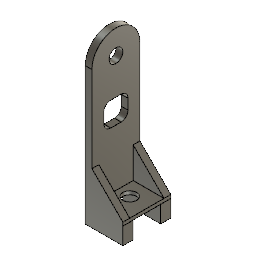
final_gear_mount v11 (Autodesk Fusion 360 design; units mm, degrees)
Autodesk Fusion 360 part; units mm, degrees
note: some values were not read from the file. Set by a fixed rule: which sketch regions a step uses.
sketch "Sketch1" plane through (0, 0, 0) normal (0, 0, 1) x (1, 0, 0)
  line L0 (0, 0) -> (11, 0)
  line L1 (11, 0) -> (11, 5)
  line L2 (11, 5) -> (0, 5)
  line L3 (0, 5) -> (0, 0)
  line L4 (1, 5) -> (10, 5)
  line L5 (10, 5) -> (10, 1)
  line L6 (10, 1) -> (1, 1)
  line L7 (1, 1) -> (1, 5)
  dimension "d1" = 1
  dimension "d2" = 1
  dimension "d3" = 1
  dimension "d4" = 9
  dimension "d5" = 4
  constraint horizontal L0
  constraint vertical L1
  constraint horizontal L2
  constraint vertical L3
  constraint coincident L0.start L3.end
  constraint horizontal L4
  constraint vertical L5
  constraint horizontal L6
  constraint vertical L7
  constraint coincident L2 L4.start
  measures "d1" distance of L3 L7
  measures "d2" distance of L1 L5
  measures "d3" distance of L0 L6
  measures "d4" distance of L5 L7
  measures "d5" distance of L2 L6
extrude "Extrude1" add sketch "Sketch1" along normal blind 95.39 contours L0 L1 L2 L3 L5 L6 L7
sketch "Sketch2" plane through (0, 1, 0) normal (0, 1, 0) x (-1, 0, 0)
  line L0 (-10, 0) -> (-1, 0)
  line L1 (-1, 0) -> (-1, 95.39)
  line L2 (-1, 95.39) -> (-10, 95.39)
  line L3 (-10, 95.39) -> (-10, 0)
  line L4 (0, 0) -> (-11, 0)
  line L5 (-11, 0) -> (-11, 1)
  line L6 (-11, 1) -> (0, 1)
  line L7 (0, 1) -> (0, 0)
  dimension "d8" = 1
  constraint horizontal L4
  constraint vertical L5
  constraint horizontal L6
  constraint vertical L7
  constraint coincident L4.start L7.end
  measures "d8" distance of L4 L6
extrude "Extrude2" add sketch "Sketch2" along normal blind 6 from surface at 4 contours L0 L1 L3 L4 L6 | L3 L4 L5 L6 | L1 L4 L6 L7
extrude "Extrude3" add 1 faces at (7, 5, 0.6667) along direction (0, -1, 0) up to surface (4 mm away)
sketch "Sketch3" plane through (0, 0, 1) normal (0, 0, 1) x (-1, 0, 0)
  line L0 (-10, -5) -> (-11, -5)
  line L1 (-11, -5) -> (-11, -11)
  line L2 (-11, -11) -> (0, -11)
  line L3 (0, -11) -> (0, -5)
  line L4 (0, -5) -> (-1, -5)
  line L5 (-1, -5) -> (-1, -1)
  line L6 (-1, -1) -> (-10, -1)
  line L7 (-10, -1) -> (-10, -5)
  line L8 (0, -7.5) -> (-11, -7.5)
  circle A0 centre (-5.5, -7.5) radius 2
  circle A1 centre (-5.5, -7.5) radius 3.5
  line L9 (0, -7.5) -> (-11, -7.5)
  line L10 (-11, -7.5) -> (-11, -14)
  line L11 (-11, -14) -> (0, -14)
  line L12 (0, -14) -> (0, -7.5)
  line L13 (-5.5, -7.5) -> (-5.5, -11)
  line L14 (-5.5, -11) -> (-5.5, -14)
  point P0 (-2, -7.5)
  dimension "d14" = 4
  dimension "d15" = 7
  dimension "d17" = 3
  dimension "d32" = 6.5
  constraint coincident L3 L8.start
  constraint coincident L1 L8.end
  constraint perpendicular L1 L8
  constraint midpoint L8 A0.centre
  constraint concentric A0 A1
  constraint coincident L8 P0
  constraint coincident A1 P0
  constraint horizontal L9
  constraint vertical L10
  constraint horizontal L11
  constraint vertical L12
  constraint coincident A0.centre A1.centre
  constraint coincident A1 L13.end
  constraint perpendicular L2 L13
  constraint midpoint L11 L14.end
  constraint perpendicular L11 L14
  measures "d14" diameter of A0
  measures "d15" diameter of A1
  measures "d17" distance of L13.end L14.end
  measures "d32" distance of L6 L9
extrude "Extrude4" add sketch "Sketch3" against normal up to surface (1 mm away) contours L1 L2 L8 A1 L9 L10 | L2 L10 L11 L14 | L2 L3 L8 A1 L9 L12 | L2 L11 L12 L14
extrude "Extrude5" cut sketch "Sketch3" against normal blind 5 contours L8 A0 L9 | L8 A0 L9 L13 | L8 A0 L9 L13
sketch "Sketch4" plane through (0, 0, 0) normal (-1, 0, 0) x (0, -1, 0)
  line L0 (-14, 0) -> (0, 0)
  line L1 (0, 0) -> (0, 95.39)
  line L2 (0, 95.39) -> (-5, 95.39)
  line L3 (-5, 95.39) -> (-5, 1)
  line L4 (-5, 1) -> (-14, 1)
  line L5 (-14, 1) -> (-14, 0)
  line L6 (-14, 1) -> (-5, 10)
  line L7 (-14, 1) -> (-7.5, 1)
  dimension "d22" = 45
  constraint coincident L4.end L5.start
  constraint coincident L3 L6.end
  measures "d22" angle of L6 L7
extrude "Extrude6" add sketch "Sketch4" against normal up to surface (1 mm away) contours L3 L4 L6 L7
ref_plane "WorkPlane1" through (5.5, 0, 0) normal (1, 0, 0) x (0, 1, 0)
mirror "Mirror1" about plane through (5.5, 0, 0) normal (1, 0, 0) of "Extrude6"
sketch "Sketch5" plane through (0, 0, 0) normal (0, 0, -1) x (1, 0, 0)
  circle A0 centre (5.5, -7.5) radius 2
  line L0 (11, -14) -> (11, 0)
  line L1 (11, 0) -> (0, 0)
  line L2 (0, 0) -> (0, -14)
  line L3 (0, -14) -> (11, -14)
  line L4 (0, 0) -> (11, 0)
  line L5 (11, 0) -> (11, -3)
  line L6 (11, -3) -> (0, -3)
  line L7 (0, -3) -> (0, 0)
  line L8 (0, -14) -> (11, -14)
  line L9 (11, -14) -> (11, -11)
  line L10 (11, -11) -> (0, -11)
  line L11 (0, -11) -> (0, -14)
  dimension "d28" = 3
  dimension "d29" = 3
  constraint horizontal L4
  constraint vertical L5
  constraint horizontal L6
  constraint vertical L7
  constraint coincident L0 L5.end
  constraint coincident L1.end L2.start
  constraint horizontal L8
  constraint vertical L9
  constraint horizontal L10
  constraint vertical L11
  constraint coincident L0 L9.end
  constraint coincident L2.end L3.start
  measures "d28" distance of L2.end L10.end
  measures "d29" distance of L4 L6
extrude "Extrude7" add sketch "Sketch5" along normal blind 5 contours L0 L2 L3 L8 L9 L10 L11 | L0 L1 L2 L4 L5 L6 L7
sketch "Sketch6" plane through (11, 0, 0) normal (1, 0, 0) x (0, 1, 0)
  line L0 (0, 0) -> (3, 0)
  line L1 (3, 0) -> (11, 0)
  line L2 (11, 0) -> (14, 0)
  line L3 (14, 0) -> (14, 1)
  line L4 (14, 1) -> (5, 10)
  line L5 (5, 10) -> (5, 95.39)
  line L6 (5, 95.39) -> (0, 95.39)
  line L7 (0, 95.39) -> (0, 0)
  line L8 (14, 1) -> (-30, 1)
  line L9 (-30, 1) -> (-30, 130)
  line L10 (-30, 130) -> (14, 130)
  line L11 (14, 130) -> (14, 1)
  constraint horizontal L8
  constraint vertical L9
  constraint horizontal L10
  constraint vertical L11
  constraint coincident L3.end L4.start
extrude "Extrude8" cut sketch "Sketch6" against normal blind 100 contours L4 L5 L6 L7 L8
sketch "Sketch7" plane through (0, 0, 1) normal (0, 0, 1) x (-1, 0, 0)
  line L0 (-11, -14) -> (0, -14)
  line L1 (0, -14) -> (0, 0)
  line L2 (0, 0) -> (-11, 0)
  line L3 (-11, 0) -> (-11, -14)
  circle A0 centre (-5.5, -7.5) radius 2
  line L4 (0, -14) -> (-2, -14)
  line L5 (-2, -14) -> (-2, 0)
  line L6 (-2, 0) -> (0, 0)
  line L7 (0, 0) -> (0, -14)
  point P0 (0, -11)
  dimension "d35" = 2
  constraint horizontal L4
  constraint vertical L5
  constraint horizontal L6
  constraint vertical L7
  constraint coincident L2 L5.end
  constraint coincident L0.end L1.start
  measures "d35" distance of L5 P0
extrude "Extrude9" add sketch "Sketch7" along normal blind 41 contours L0 L1 L2 L4 L5 L6 L7
sketch "Sketch8" plane through (0, 0, 0) normal (-1, 0, 0) x (0, -1, 0)
  line L0 (-14, 42) -> (-14, -5)
  line L1 (-14, -5) -> (-11, -5)
  line L2 (-11, -5) -> (-11, 0)
  line L3 (-11, 0) -> (-3, 0)
  line L4 (-3, 0) -> (-3, -5)
  line L5 (-3, -5) -> (0, -5)
  line L6 (0, -5) -> (0, 42)
  line L7 (0, 42) -> (-14, 42)
  line L8 (-7, 42) -> (-7, 26)
  circle A0 centre (-7, 35) radius 7
  circle A1 centre (-7, 35) radius 2
  dimension "d38" = 4
  constraint midpoint L7 L8.start
  constraint perpendicular L7 L8
  constraint coincident L8 A0.centre
  constraint coincident L8.start A0
  constraint tangent L6 A0
  constraint concentric A0 A1
  measures "d38" diameter of A1
extrude "Extrude10" cut sketch "Sketch8" against normal blind 10 contours L0 L7 A0 | L6 L7 A0 | L8 A1 | L8 A1
sketch "Sketch9" plane through (2, 0, 0) normal (1, 0, 0) x (0, 1, 0)
  arc A0 (14, 35) -> (0, 35) centre (7, 35) ccw
  line L0 (0, 35) -> (0, 1)
  line L1 (0, 1) -> (14, 1)
  line L2 (14, 1) -> (14, 35)
  circle A1 centre (7, 35) radius 2
  line L3 (4.5, 18.5) -> (9.5, 18.5)
  line L4 (9.5, 18.5) -> (9.5, 22.5)
  line L5 (9.5, 22.5) -> (4.5, 22.5)
  line L6 (4.5, 22.5) -> (4.5, 18.5)
  line L7 (7, 22.5) -> (7, 35)
  dimension "d41" = 5
  dimension "d42" = 4
  dimension "d43" = 90
  dimension "d44" = 12.5
  constraint horizontal L3
  constraint vertical L4
  constraint horizontal L5
  constraint vertical L6
  constraint midpoint L5 L7.start
  constraint coincident A0.centre A1.centre
  measures "d41" distance of L3.start L3.end
  measures "d42" distance of L3.end L4.end
  measures "d43" angle of L5 L7
  measures "d44" distance of L7.start A0.centre
extrude "Extrude11" cut sketch "Sketch9" against normal blind 10 contours L3 L4 L5 L6
extrude "Extrude12" cut 1 faces at (1.3333, 7.8333, 22.5) along direction (0, 0, 1) blind 1
sketch "Sketch10" plane through (0, 0, 0) normal (-1, 0, 0) x (0, -1, 0)
  line L0 (-4.5, 23.5) -> (-4.5, 18.5)
  line L1 (-4.5, 18.5) -> (-9.5, 18.5)
  line L2 (-9.5, 18.5) -> (-9.5, 23.5)
  line L3 (-9.5, 23.5) -> (-4.5, 23.5)
  circle A0 centre (-7, 35) radius 2
  arc A1 (0, 35) -> (-14, 35) centre (-7, 35) ccw
  line L4 (-14, 35) -> (-14, -5)
  line L5 (-14, -5) -> (-11, -5)
  line L6 (-11, -5) -> (-11, 0)
  line L7 (-11, 0) -> (-3, 0)
  line L8 (-3, 0) -> (-3, -5)
  line L9 (-3, -5) -> (0, -5)
  line L10 (0, -5) -> (0, 35)
  line L11 (-5.5, 17.5) -> (-8.5, 17.5)
  line L12 (-10.5, 19.5) -> (-10.5, 22.5)
  line L13 (-8.5, 24.5) -> (-5.5, 24.5)
  line L14 (-3.5, 22.5) -> (-3.5, 19.5)
  arc A2 (-8.5, 24.5) -> (-10.5, 22.5) centre (-8.5, 22.5) ccw
  arc A3 (-3.5, 22.5) -> (-5.5, 24.5) centre (-5.5, 22.5) ccw
  arc A4 (-5.5, 17.5) -> (-3.5, 19.5) centre (-5.5, 19.5) ccw
  arc A5 (-10.5, 19.5) -> (-8.5, 17.5) centre (-8.5, 19.5) ccw
  dimension "d50" = 2
  constraint parallel L1 L11
  constraint parallel L2 L12
  constraint parallel L3 L13
  constraint parallel L0 L14
  constraint tangent L12 A2
  constraint tangent L13 A2
  constraint tangent L13 A3
  constraint tangent L14 A3
  constraint equal A2 A3
  constraint tangent L11 A4
  constraint tangent L14 A4
  constraint equal A2 A4
  constraint tangent L11 A5
  constraint tangent L12 A5
  constraint equal A2 A5
  measures "d50" radius of A2
extrude "Extrude13" cut sketch "Sketch10" against normal blind 5 contours L11 L12 L13 L14 A2 A3 A4 A5
sketch "Sketch11" plane through (0, 0, 0) normal (0, -1, 0) x (1, 0, 0)
  line L0 (2, 35) -> (0, 35)
  line L1 (0, 35) -> (0, -5)
  line L2 (0, -5) -> (11, -5)
  line L3 (11, -5) -> (11, 0)
  line L4 (11, 0) -> (11, 1)
  line L5 (11, 1) -> (2, 1)
  line L6 (2, 1) -> (2, 35)
  line L7 (11, 1) -> (2, 10)
  dimension "d53" = 45
  constraint coincident L4.end L5.start
  constraint coincident L6 L7.end
  measures "d53" angle of L5 L7
extrude "Extrude14" add sketch "Sketch11" against normal up to surface (14 mm away) contours L5 L6 L7
sketch "Sketch12" plane through (11, 0, 0) normal (1, 0, 0) x (0, 1, 0)
  line L0 (14, 1) -> (0, 1)
  line L1 (0, 1) -> (0, 0)
  line L2 (0, 0) -> (3, 0)
  line L3 (3, 0) -> (11, 0)
  line L4 (11, 0) -> (14, 0)
  line L5 (14, 0) -> (14, 1)
  line L6 (2, 0) -> (12, 0)
  line L7 (12, 0) -> (12, 12)
  line L8 (12, 12) -> (2, 12)
  line L9 (2, 12) -> (2, 0)
  dimension "d57" = 2
  dimension "d58" = 2
  constraint horizontal L6
  constraint vertical L7
  constraint horizontal L8
  constraint vertical L9
  measures "d57" distance of L1 L9
  measures "d58" distance of L5 L7
extrude "Extrude15" cut sketch "Sketch12" against normal up to surface (9 mm away) contours L0 L7 L8 L9
